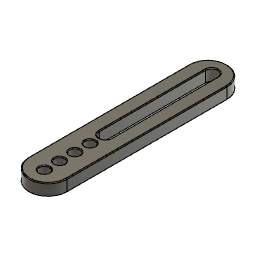
B914F (Autodesk Fusion 360 design; units mm, degrees)
Autodesk Fusion 360 part; units mm, degrees
sketch "Esboço1" plane through (0, 0, 0) normal (0, 1, 0) x (1, 0, 0)
  line L0 (15.7988, 74.5632) -> (15.7988, 7.8598)
  line L1 (0, 7.8598) -> (0, 74.5632)
  circle A0 centre (7.8994, 6.35) radius 2.108
  circle A1 centre (7.8994, 12.7) radius 2.108
  circle A2 centre (7.8994, 19.05) radius 2.108
  circle A3 centre (7.8994, 25.4) radius 2.108
  line L2 (7.8994, 29.21) -> (7.8994, 31.75)
  arc A4 (15.7988, 74.4838) -> (0, 74.4838) centre (7.8994, 74.5235) ccw
  arc A5 (0, 7.9392) -> (15.7988, 7.9392) centre (7.8994, 7.8995) ccw
  arc A6 (5.3594, 31.75) -> (10.4394, 31.75) centre (7.8994, 31.75) ccw
  arc A7 (10.4394, 76.073) -> (5.3594, 76.073) centre (7.8994, 76.073) ccw
  line L3 (5.3594, 31.75) -> (5.3594, 76.073)
  line L4 (10.4394, 31.75) -> (10.4394, 76.073)
  dimension "d4" = 6.35
  dimension "d5" = 6.35
  dimension "d6" = 6.35
  dimension "d8" = 5.08
  dimension "d11" = 4.216
  dimension "d12" = 4.216
  dimension "d13" = 4.216
  dimension "d14" = 4.216
  dimension "d15" = 6.35
  dimension "d16" = 5.08
  constraint coincident L2.end A6.centre
  constraint coincident L0.start A4
  constraint coincident L1.end A4
  constraint coincident L1 A4.end
  constraint coincident L0 A4.start
  constraint coincident L0.end A5
  constraint coincident L1.start A5
  constraint coincident L0 A5.end
  constraint coincident L1 A5.start
  constraint coincident L2.start A6
  constraint tangent A6 L3
  constraint tangent A7 L4
  measures "d4" distance of A0.centre A1.centre
  measures "d5" distance of A1.centre A2.centre
  measures "d6" distance of A2.centre A3.centre
  measures "d8" diameter of A7
  measures "d11" diameter of A0
  measures "d12" diameter of A1
  measures "d13" diameter of A2
  measures "d14" diameter of A3
  measures "d15" distance of A3.centre L2.end
  measures "d16" diameter of A6
extrude "Extrusão1" add sketch "Esboço1" along normal blind 4.7752
chamfer "Chanfro1" distance 0.3 angle 45 12 edges at (15.7988, 4.7752, -41.2115) (7.8994, 4.7752, 0) (0, 4.7752, -41.2115) (7.8994, 4.7752, -82.423) (10.4394, 4.7752, -53.9115) (7.8994, 4.7752, -29.21) (5.3594, 4.7752, -53.9115) (7.8994, 4.7752, -78.613) (5.9341, 4.7752, -26.1623) (5.9341, 4.7752, -19.8123) (5.9341, 4.7752, -13.4623) (5.9341, 4.7752, -7.1123)
